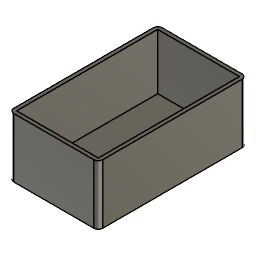
Simple Box enclosure (Autodesk Fusion 360 design; units mm, degrees)
part number: 2026-06-27-11-58-38-575
Autodesk Fusion 360 part; units mm, degrees
sketch "Sketch1" plane through (0, 0, 0) normal (0, 0, 1) x (1, 0, 0)
  line L0 (30, -50) -> (-30, -50)
  line L1 (-30, -50) -> (-30, 50)
  line L2 (-30, 50) -> (30, 50)
  line L3 (30, 50) -> (30, -50)
  line L4 (30, -50) -> (-30, 50) construction
  line L5 (-30, -50) -> (30, 50) construction
  dimension "d1" = 60
  dimension "d2" = 100
  constraint horizontal L0
  constraint perpendicular L0 L1
  constraint parallel L0 L2
  constraint parallel L1 L3
  constraint coincident L4 origin
  constraint coincident L5 origin
  measures "d1" distance of L1.end L2.end
  measures "d2" distance of L0.end L1.end
extrude "Extrude1" add sketch "Sketch1" along normal blind 40
shell "Shell1" thickness 2.5 removed faces 1 at (10, -16.6667, 40)
fillet "Fillet1" radius 3 4 edges at (30, 50, 20) (-30, 50, 20) (30, -50, 20) (-30, -50, 20)
